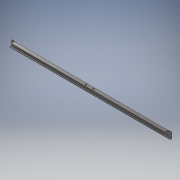
# Autodesk Inventor part: Batente Sup.
Saved by Autodesk Inventor 2017 (Build 210142000, 142)
## iProperties
Created: 2019-06-18
Part Number: Batente Sup.
Material: Stainless Steel
Document SubType Name: Sheet Metal
Designer: leonardo.prado
Density: 8 g/cm^3
Sheet Metal Rule: Default_mm
Appearance: Semi-Polished
Description: Chapa de Aço Inox Aisi 304 - #1,5mm
Mass: 572.804 g
Surface Area: 982.315 cm^2
Volume: 71.6005 cm^3
Flat Pattern Width: 5.62858 cm
Flat Pattern Length: 86.0598 cm
Flat Pattern Area: 484.395 cm^2
Sheet Metal Width: 56,286 mm
Sheet Metal Length: 860,598 mm
Sheet Metal Area: 48439,481 mm^2
Author: leonardo.prado
Comments: 56 x 860
Autodesk Inventor part; units mm, degrees
ref_plane "YZ Plane" through (0, 0, 0) normal (1, 0, 0) x (0, 1, 0)
ref_plane "XZ Plane" through (0, 0, 0) normal (0, 1, 0) x (-1, 0, 0)
ref_plane "XY Plane" through (0, 0, 0) normal (0, 0, 1) x (1, 0, 0)
sketch "Sketch2" plane through (0, 0, 0) normal (0, 1, 0) x (-1, 0, 0)
  line L0 (-430.299, 15) -> (430.299, 15)
  line L1 (430.299, 15) -> (430.299, -15)
  line L2 (430.299, -15) -> (-430.299, -15)
  line L3 (-430.299, -15) -> (-430.299, 15)
  line L4 (-430.299, 15) -> (430.299, -15) construction
  line L5 (430.299, 15) -> (-430.299, -15) construction
  point P0 (0, 0)
  dimension "d12" = 860.598
  dimension "d13" = 30
  measures "d12" distance of L1.end L2.end
  measures "d13" distance of L0.end L1.end
extrude "Plate2" add sketch "Sketch2" along normal blind 1.5
sketch "Sketch3" plane through (-430.299, 0, 15) normal (0, 0, 1) x (1, 0, 0)
  line L0 (842.098, 0) -> (18.5, 0)
  line L1 (18.5, 0) -> (18.5, -18.5)
  line L2 (18.5, -18.5) -> (842.098, -18.5)
  line L3 (842.098, -18.5) -> (842.098, 0)
  constraints: 8 end point
edge flange "Flange1" height 20 angle 90 thickness 1.5 bend radius 1.5 thickness toward (0, 0, 1) relief straight relief width 1.5 relief depth 0.75 edges at (0, 0, 15) wall of the first edge with corners at (411.799, 0, 15) (-411.799, 0, 15) (-411.799, -18.5, 15) (411.799, -18.5, 15)
bend "Bend2"
corner "Corner2"
sketch "Sketch4" plane through (430.299, 1.5, -13.5) normal (0, 0, -1) x (-1, 0, 0)
  line L0 (860.598, 0) -> (0, 0)
  line L1 (0, 0) -> (0, -10)
  line L2 (0, -10) -> (860.598, -10)
  line L3 (860.598, -10) -> (860.598, 0)
  constraints: 6 end point, 1 horizontal, 1 perpendicular, 1 vertical
edge flange "Flange2" height 10 angle 90 thickness 1.5 bend radius 1.5 thickness toward (0, 0, -1) relief straight relief width 1.5 relief depth 0.75 edges at (0, 0, -15) wall of the first edge with corners at (-430.299, 1.5, -13.5) (430.299, 1.5, -13.5) (430.299, -8.5, -13.5) (-430.299, -8.5, -13.5)
bend "Bend3"
corner "Corner3"
sketch "Sketch5" plane through (411.799, -18.5, 15) normal (0, 0, -1) x (-1, 0, 0)
  circle A0 centre (391.799, 8.5) radius 2.067 construction
  circle A1 centre (431.799, 8.5) radius 2.067 construction
  circle A2 centre (391.799, 8.5) radius 2.75
  circle A3 centre (431.799, 8.5) radius 2.75
  point P0 (411.799, 18.5)
  dimension "d36" = 5.5
  dimension "d37" = 5.5
  constraints: 2 centre point, 2 coincident
  measures "d36" diameter of A2
  measures "d37" diameter of A3
extrude "Extrusion1" cut sketch "Sketch5" against normal blind 1.5
chamfer "Chamfer1" distance 1.5 angle 45 2 edges at (22.75, -10, 16.5) (-17.25, -10, 16.5)
equation "\"d38\" = Thickness"
equation "\"d15\" = BendReliefWidth"
equation "\"d16\" = BendReliefDepth"
equation "\"d17\" = MinimumRemnant"
equation "\"d18\" = BendRadius"
equation "\"d22\" = BendRadius"
equation "\"d23\" = CornerReliefSize"
equation "\"d24\" = GapSize"
equation "\"d25\" = JacobiRadiusSize"
equation "\"d26\" = BendReliefWidth"
equation "\"d27\" = BendReliefDepth"
equation "\"d28\" = MinimumRemnant"
equation "\"d29\" = BendRadius"
equation "\"d32\" = BendRadius"
equation "\"d33\" = CornerReliefSize"
equation "\"d34\" = GapSize"
equation "\"d35\" = JacobiRadiusSize"
equation "\"BendRadius\" = Thickness"
equation "\"BendReliefWidth\" = Thickness"
equation "\"BendReliefDepth\" = 0.5 * Thickness"
equation "\"CornerReliefSize\" = 4 * Thickness"
equation "\"MinimumRemnant\" = 2 * Thickness"
equation "\"TransitionRadius\" = BendRadius"
equation "\"JacobiRadiusSize\" = BendRadius"
equation "\"GapSize\" = Thickness"
equation "\"d14\" = BendRadius"
equation "\"Thickness\" = 1.5"
body "Solid2"
